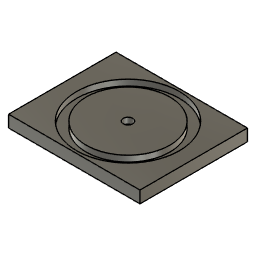
sand_cube_back (Autodesk Fusion 360 design; units mm, degrees)
Autodesk Fusion 360 part; units mm, degrees
note: some values were not read from the file. Set by a fixed rule: which sketch regions a step uses.
sketch "Sketch1" plane through (0, 0, 0) normal (0, 0, 1) x (1, 0, 0)
  line L0 (0, 0) -> (55, 0)
  line L1 (55, 0) -> (55, 45)
  line L2 (55, 45) -> (0, 45)
  line L3 (0, 45) -> (0, 0)
  dimension "d1" = 55
  dimension "d2" = 45
  constraint horizontal L0
  constraint vertical L1
  constraint horizontal L2
  constraint vertical L3
  constraint coincident L0.start L3.end
  measures "d1" distance of L0.start L0.end
  measures "d2" distance of L0.start L2.end
extrude "Extrude1" add sketch "Sketch1" along normal blind 5
sketch "Sketch2" plane through (0, 0, 5) normal (0, 0, 1) x (-1, 0, 0)
  line L0 (0, -45) -> (0, 0)
  line L1 (0, 0) -> (-55, 0)
  line L2 (-55, 0) -> (-55, -45)
  line L3 (-55, -45) -> (0, -45)
  line L4 (0, -45) -> (-55, -45)
  line L5 (-55, -45) -> (-55, -50)
  line L6 (-55, -50) -> (0, -50)
  line L7 (0, -50) -> (0, -45)
  line L8 (0, 0) -> (-55, 0)
  line L9 (-55, 0) -> (-55, 5)
  line L10 (-55, 5) -> (0, 5)
  line L11 (0, 5) -> (0, 0)
  line L12 (0, -50) -> (-55, 5)
  line L13 (-55, -50) -> (0, 5)
  circle A0 centre (-27.5, -22.5) radius 2
  circle A1 centre (-27.5, -22.5) radius 17.5
  circle A2 centre (-27.5, -22.5) radius 21.5
  dimension "d5" = 55
  dimension "d6" = 5
  dimension "d7" = 55
  dimension "d8" = 5
  dimension "d9" = 4
  dimension "d10" = 35
  dimension "d11" = 43
  constraint horizontal L4
  constraint vertical L5
  constraint horizontal L6
  constraint vertical L7
  constraint coincident L0.start L3.end
  constraint horizontal L8
  constraint vertical L9
  constraint horizontal L10
  constraint vertical L11
  constraint coincident L0.end L1.start
  constraint midpoint L13 A0.centre
  constraint concentric A0 A1
  constraint concentric A0 A2
  measures "d5" distance of L0.start L2.end
  measures "d6" distance of L0.start L6.end
  measures "d7" distance of L0.end L1.end
  measures "d8" distance of L0.end L10.end
  measures "d9" diameter of A0
  measures "d10" diameter of A1
  measures "d11" diameter of A2
extrude "Extrude2" cut sketch "Sketch2" against normal blind 2.5 contours L12 L13 A1 A2 | L12 L13 A1 A2 | L12 L13 A1 A2 | L12 L13 A1 A2 | L12 L13 A0 | L12 L13 A0 | L12 L13 A0 | L12 L13 A0
